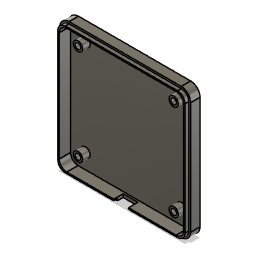
enclosure.bottom.v4 (Autodesk Fusion 360 design; units mm, degrees)
Autodesk Fusion 360 part; units mm, degrees
sketch "Sketch2" plane through (0, 1.6535, 0) normal (0, 1, 0) x (-1, 0, 0)
  line L0 (-63.6703, 1) -> (-5.6703, 1)
  line L1 (-5.6703, 1) -> (-5.6703, 7)
  line L2 (-5.6703, 7) -> (-63.6703, 7)
  line L3 (-63.6703, 7) -> (-63.6703, 1)
  line L4 (-30.5955, 7) -> (-38.4299, 7)
  line L5 (-38.4299, 7) -> (-38.4299, 2)
  line L6 (-38.4299, 2) -> (-30.5955, 2)
  line L7 (-30.5955, 2) -> (-30.5955, 7)
  dimension "d1" = 5
  constraint horizontal L4
  constraint vertical L5
  constraint horizontal L6
  constraint vertical L7
  constraint coincident L2 L4.start
  measures "d1" distance of L4.end L5.end
sketch "Sketch3" plane through (0, 0, 1) normal (0, 0, 1) x (1, 0, 0)
  circle A0 centre (9.6172, 60.4797) radius 2.5
  circle A1 centre (60.4172, 9.6797) radius 2.5
  circle A2 centre (9.6172, 9.6797) radius 2.5
  circle A3 centre (60.4172, 60.4797) radius 2.5
  line L0 (68.4203, 4.9035) -> (68.4203, 64.4035)
  arc A4 (68.4203, 64.4035) -> (64.4203, 68.4035) centre (64.4203, 64.4035) ccw
  line L1 (64.4203, 68.4035) -> (4.9203, 68.4035)
  arc A5 (4.9203, 68.4035) -> (0.9203, 64.4035) centre (4.9203, 64.4035) ccw
  line L2 (0.9203, 64.4035) -> (0.9203, 4.9035)
  arc A6 (0.9203, 4.9035) -> (4.9203, 0.9035) centre (4.9203, 4.9035) ccw
  line L3 (4.9203, 0.9035) -> (64.4203, 0.9035)
  arc A7 (64.4203, 0.9035) -> (68.4203, 4.9035) centre (64.4203, 4.9035) ccw
  line L4 (5.6703, 67.6535) -> (63.6703, 67.6535)
  line L5 (67.6703, 63.6535) -> (67.6703, 5.6535)
  line L6 (63.6703, 1.6535) -> (5.6703, 1.6535)
  line L7 (1.6703, 5.6535) -> (1.6703, 63.6535)
  arc A8 (5.6703, 67.6535) -> (1.6703, 63.6535) centre (5.6703, 63.6535) ccw
  arc A9 (67.6703, 63.6535) -> (63.6703, 67.6535) centre (63.6703, 63.6535) ccw
  arc A10 (63.6703, 1.6535) -> (67.6703, 5.6535) centre (63.6703, 5.6535) ccw
  arc A11 (1.6703, 5.6535) -> (5.6703, 1.6535) centre (5.6703, 5.6535) ccw
  dimension "d2" = 4
  dimension "d3" = 0.75
  dimension "d4" = 0.75
  dimension "d5" = 0.75
  dimension "d6" = 0.75
  constraint horizontal L4
  constraint vertical L5
  constraint horizontal L6
  constraint vertical L7
  constraint tangent L7 A8
  constraint tangent L4 A8
  constraint tangent L4 A9
  constraint tangent L5 A9
  constraint equal A8 A9
  constraint tangent L5 A10
  constraint tangent L6 A10
  constraint equal A8 A10
  constraint tangent L7 A11
  constraint tangent L6 A11
  constraint equal A8 A11
  measures "d2" radius of A8
  measures "d3" distance of L2 L7
  measures "d4" distance of L3 L6
  measures "d5" distance of L0 L5
  measures "d6" distance of L1 L4
sketch "Sketch1" plane through (0, 0, 0) normal (0, 0, 1) x (1, 0, 0)
  circle A0 centre (9.6172, 9.6797) radius 1.5
  circle A1 centre (60.4172, 9.6797) radius 1.5
  arc A2 (4.9203, 69.4035) -> (-0.0797, 64.4035) centre (4.9203, 64.4035) ccw
  arc A3 (64.4203, -0.0965) -> (69.4203, 4.9035) centre (64.4203, 4.9035) ccw
  circle A4 centre (60.4172, 60.4797) radius 1.5
  line L0 (-6, 9.6797) -> (72, 9.6797) construction
  line L1 (35.0172, 92) -> (35.0172, -8) construction
  line L2 (64.4203, 69.4035) -> (4.9203, 69.4035)
  line L3 (60.4172, -4) -> (60.4172, 71) construction
  line L4 (-7, 60.4797) -> (90.0735, 60.4797) construction
  arc A5 (69.4203, 64.4035) -> (64.4203, 69.4035) centre (64.4203, 64.4035) ccw
  line L5 (4.9203, -0.0965) -> (64.4203, -0.0965)
  line L6 (-7, 66.8297) -> (83, 66.8297) construction
  arc A6 (-0.0797, 4.9035) -> (4.9203, -0.0965) centre (4.9203, 4.9035) ccw
  line L7 (-0.0797, 64.4035) -> (-0.0797, 4.9035)
  line L8 (-5, 3.3297) -> (86.8002, 3.3297) construction
  line L9 (9.6172, 82) -> (9.6172, -14) construction
  line L10 (69.4203, 4.9035) -> (69.4203, 64.4035)
  circle A7 centre (9.6172, 60.4797) radius 1.5
  point P0 (2.2672, 67.8297)
  point P1 (67.7672, 67.8297)
  point P2 (69.4203, -0.0965)
  point P3 (69.4203, 69.4035)
  point P4 (-0.0797, 69.4035)
  dimension "d138" = 69.5
  dimension "d139" = 69.5
  dimension "d140" = 65.5
  dimension "d143" = 6.35
  dimension "d144" = 6.35
  dimension "d156" = 3
  dimension "d158" = 3
  dimension "d160" = 3
  dimension "d162" = 3
  dimension "d164" = 5
  dimension "d165" = 5
  dimension "d166" = 5
  dimension "d167" = 5
  constraint horizontal L5
  constraint vertical L10
  constraint horizontal L2
  constraint vertical L7
  constraint tangent A6 L7
  constraint tangent L5 A6
  constraint coincident P2 L5
  constraint coincident P2 L10
  constraint tangent A3 L5
  constraint tangent A3 L10
  constraint coincident P3 L2
  constraint coincident P3 L10
  constraint tangent L2 A5
  constraint tangent A5 L10
  constraint coincident P4 L7
  constraint coincident P4 L2
  constraint tangent A2 L7
  constraint tangent A2 L2
  constraint horizontal L6
  constraint horizontal L8
  constraint perpendicular L5 L9
  constraint perpendicular L2 L3
  measures "d138" distance of P2 P3
  measures "d139" distance of P3 P4
  measures "d140" distance of P0 P1
  measures "d143" distance of L0 L8
  measures "d144" distance of L4 L6
  measures "d156" diameter of A7
  measures "d158" diameter of A4
  measures "d160" diameter of A1
  measures "d162" diameter of A0
  measures "d164" radius of A2
  measures "d165" radius of A5
  measures "d166" radius of A3
  measures "d167" radius of A6
extrude "Extrude1" add sketch "Sketch1" along normal blind 5
shell "Shell1" thickness 1 removed faces 1 at (26.9171, 26.9532, 5)
extrude "Extrude3" add sketch "Sketch3" along normal blind 6 contours L0 A4 L1 A5 L2 A6 L3 A7
hole "Hole2" at (60.4172, 60.4797, 0) direction (0, 0, 1) diameter 3 depth 3 tip angle 118 countersink diameter 7 countersink angle 120
hole "Hole10" at (60.4172, 9.6797, 0) direction (0, 0, 1) diameter 3 depth 2.75 tip angle 118 countersink diameter 7 countersink angle 120
hole "Hole11" at (9.6172, 9.6797, 0) direction (0, 0, 1) diameter 3 depth 2.75 tip angle 118 countersink diameter 7 countersink angle 120
hole "Hole12" at (9.6172, 60.4797, 0) direction (0, 0, 1) diameter 3 depth 2.75 tip angle 118 countersink diameter 7 countersink angle 120
extrude "Extrude4" cut sketch "Sketch2" against normal blind 2 contours L2 L4 L5 L6 L7
equation "d143 = mount_post_offset"
equation "d144 = mount_post_offset"
equation "d156 = mount_post_pcb_holder"
equation "d158 = mount_post_pcb_holder"
equation "d160 = mount_post_pcb_holder"
equation "d162 = mount_post_pcb_holder"
equation "d164 = shell_corner_radius"
equation "d165 = shell_corner_radius"
equation "d166 = shell_corner_radius"
equation "d167 = shell_corner_radius"
equation "mount_post_offset = 6.35 mm"
equation "mount_post_pcb_holder = 3 mm"
equation "shell_corner_radius = 5 mm"
